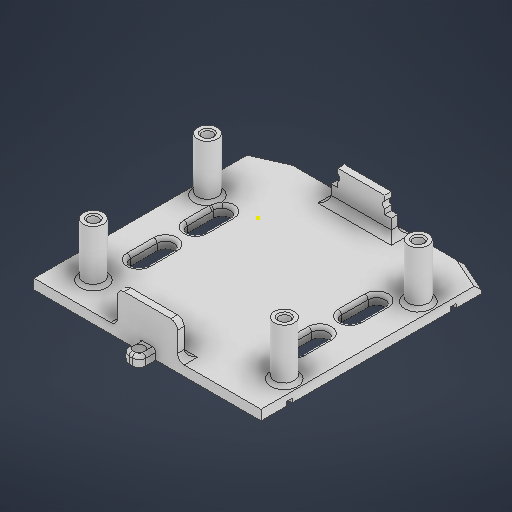
# Autodesk Inventor part: Podstawa2
Saved by Autodesk Inventor 2026 (Build 300175000, 175)
## iProperties
Created: 2025-04-23
Part Number: Podstawa2
Material: Generic
Document SubType Name: Modeling
Designer: isan
Density: 1 g/cm^3
Appearance: Default
Author: isan
Autodesk Inventor part; units mm, degrees
ref_plane "YZ Plane" through (0, 0, 0) normal (1, 0, 0) x (0, 1, 0)
ref_plane "XZ Plane" through (0, 0, 0) normal (0, 1, 0) x (-1, 0, 0)
ref_plane "XY Plane" through (0, 0, 0) normal (0, 0, 1) x (1, 0, 0)
sketch "Sketch2" plane through (0, 0, 0) normal (0, 1, 0) x (-1, 0, 0)
  line L0 (-34, 33) -> (34, 33)
  line L1 (34, 33) -> (34, -33)
  line L2 (34, -33) -> (-34, -33)
  line L3 (-34, -33) -> (-34, 33)
  line L4 (-34, 33) -> (34, -33) construction
  line L5 (34, 33) -> (-34, -33) construction
  point P0 (0, 0)
  dimension "d5" = 66
  dimension "d6" = 68
  constraints: 12 end point, 2 midpoint, 2 parallel, 1 horizontal, 1 perpendicular
  measures "d5" distance of L0.end L1.end
  measures "d6" distance of L1.end L2.end
extrude "Extrusion1" add sketch "Sketch2" along normal blind 3
sketch "Sketch3" plane through (0, 3, 0) normal (0, 1, 0) x (1, 0, 0)
  line L0 (-23.1, 12.5) -> (-23.1, 4.5) construction
  line L1 (-25.6, 12.5) -> (-25.6, 4.5)
  line L2 (-20.6, 4.5) -> (-20.6, 12.5)
  arc A0 (-20.6, 12.5) -> (-25.6, 12.5) centre (-23.1, 12.5) ccw
  arc A1 (-25.6, 4.5) -> (-20.6, 4.5) centre (-23.1, 4.5) ccw
  line L3 (-34, 33) -> (-34, -33) projected
  point P0 (0, 0)
  point P1 (-23.1, 8.5)
  point P2 (-23.1, 15)
  point P3 (-23.1, 2)
  point P4 (-25.6, 8.5)
  dimension "d9" = 13
  dimension "d12" = 2.5
  dimension "d13" = 8.4
  dimension "d14" = 2
  constraints: 8 end point, 6 point on circle, 4 tangent, 2 centre point, 2 midpoint, 1 parallel, 1 vertical
  measures "d9" distance of point (-23.1, 15) point (-23.1, 2)
  measures "d12" radius of A0
  measures "d13" distance from line of L3 point (-25.6, 8.5)
  measures "d14" vertical distance of point (0, 0) point (-23.1, 2)
extrude "Extrusion2" cut sketch "Sketch3" against normal blind 3
mirror "Mirror1" about plane through (0, 0, 0) normal (1, 0, 0) of "Extrusion2"
mirror "Mirror2" about plane through (0, 0, 0) normal (0, 0, 1) of "Extrusion2", "Mirror1"
sketch "Sketch4" plane through (0, 3, 0) normal (0, 1, 0) x (1, 0, 0)
  circle A0 centre (-29.6, 14.557) radius 3
  line L0 (-34, 33) -> (-34, -33) projected
  line L1 (-34, -33) -> (34, -33) projected
  line L2 (34, 33) -> (-34, 33) projected
  circle A1 centre (29.583, -21.6) radius 3
  line L3 (34, -33) -> (34, 33) projected
  circle A2 centre (29.525, 18.595) radius 3
  circle A3 centre (-24.6, -24.6) radius 3
  point P0 (0, 0)
  dimension "d23" = 6
  dimension "d28" = 6
  dimension "d31" = 6
  dimension "d34" = 6
  dimension "d65" = 29.6
  dimension "d66" = 14.557
  dimension "d67" = 29.525
  dimension "d68" = 18.595
  dimension "d69" = 21.6
  dimension "d70" = 29.583
  dimension "d71" = 24.6
  dimension "d72" = 24.6
  constraints: 4 centre point
  measures "d23" diameter of A0
  measures "d28" diameter of A1
  measures "d31" diameter of A2
  measures "d34" diameter of A3
  measures "d65" horizontal distance of point (0, 0) A0.centre
  measures "d66" vertical distance of point (0, 0) A0.centre
  measures "d67" horizontal distance of point (0, 0) A2.centre
  measures "d68" vertical distance of point (0, 0) A2.centre
  measures "d69" vertical distance of point (0, 0) A1.centre
  measures "d70" horizontal distance of point (0, 0) A1.centre
  measures "d71" horizontal distance of A3.centre point (0, 0)
  measures "d72" horizontal distance of point (0, 0) A3.centre
extrude "Extrusion3" add sketch "Sketch4" along normal blind 16 contours A0 | A1 | A2 | A3
sketch "Sketch5" plane through (0, 3, 0) normal (0, 1, 0) x (1, 0, 0)
  line L0 (-9, 33) -> (9, 33)
  line L1 (9, 33) -> (9, 31)
  line L2 (9, 31) -> (-9, 31)
  line L3 (-9, 31) -> (-9, 33)
  line L4 (34, 33) -> (-34, 33) projected
  point P0 (0, 0)
  point P1 (0, 33)
  dimension "d39" = 2
  dimension "d40" = 18
  constraints: 8 end point, 2 midpoint, 2 parallel, 1 collinear, 1 horizontal, 1 perpendicular
  measures "d39" distance of L0.end L1.end
  measures "d40" distance of L0.start L0.end
extrude "Extrusion4" add sketch "Sketch5" along normal blind 10
fillet "Fillet1" radius 2 5 edges at (9, 13, -32) (9, 3, -32) (0, 3, -31) (-9, 13, -32) (-9, 3, -32)
mirror "Mirror3" about plane through (0, 0, 0) normal (0, 0, 1) of "Extrusion4", "Fillet1"
sketch "Sketch6" plane through (-29.6, 19, -14.557) normal (0, 1, 0) x (1, 0, 0)
  point P0 (29.6, -14.557)
sketch "Sketch7" plane through (-29.6, 19, -14.557) normal (0, 1, 0) x (1, 0, 0)
  circle A0 centre (0, 0) radius 1.5
  circle A1 centre (0, 0) radius 3 projected
  point P0 (29.6, -14.557)
  dimension "d44" = 3
  constraints: 1 centre point, 1 coincident
  measures "d44" diameter of A0
extrude "Extrusion5" cut sketch "Sketch7" against normal blind 10 contours A0
sketch "Sketch8" plane through (29.525, 19, -18.595) normal (0, 1, 0) x (1, 0, 0)
  circle A0 centre (0, 0) radius 1.5
  point P0 (-29.525, -18.595)
  dimension "d48" = 3
  constraints: 1 centre point
  measures "d48" diameter of A0
extrude "Extrusion6" cut sketch "Sketch8" against normal blind 10
sketch "Sketch9" plane through (-24.6, 19, 24.6) normal (0, 1, 0) x (1, 0, 0)
  circle A0 centre (0, 0) radius 3 projected
  circle A1 centre (0, 0) radius 1.5
  circle A2 centre (54.183, 3) radius 1.5
  circle A3 centre (54.183, 3) radius 3 projected
  point P0 (24.6, 24.6)
  dimension "d51" = 3
  dimension "d52" = 3
  constraints: 2 centre point, 2 coincident
  measures "d51" diameter of A1
  measures "d52" diameter of A2
extrude "Extrusion7" cut sketch "Sketch9" against normal blind 10 contours A1 | A2
sketch "Sketch11" plane through (0, 0, 0) normal (0, -1, 0) x (1, 0, 0)
  line L0 (-34, 25.4) -> (-13.9, 25.4)
  line L1 (-13.9, 25.4) -> (-13.9, 23.6)
  line L2 (-13.9, 23.6) -> (-34, 23.6)
  line L3 (-34, 23.6) -> (-34, 25.4)
  line L4 (-34, -33) -> (-34, 33) projected
  line L5 (-34, 33) -> (34, 33) projected
  point P0 (0, 0)
  point P1 (-34, 24.5)
  dimension "d60" = 1.8
  dimension "d61" = 20.1
  dimension "d62" = 8.5
  constraints: 8 end point, 2 parallel, 1 collinear, 1 horizontal, 1 midpoint, 1 perpendicular
  measures "d60" distance of L0.end L1.end
  measures "d61" distance of L1.end L2.end
  measures "d62" distance from line of L5 point (-34, 24.5)
extrude "Extrusion9" cut sketch "Sketch11" against normal blind 1.2
mirror "Mirror6" about plane through (0, 0, 0) normal (1, 0, 0) of "Extrusion9"
mirror "Mirror7" about plane through (0, 0, 0) normal (0, 0, 1) of "Extrusion9", "Mirror6"
chamfer "Chamfer3" distance 0.4 angle 45 4 edges at (-31.1, 19, -14.557) (28.025, 19, -18.595) (28.083, 19, 21.6) (-26.1, 19, 24.6)
sketch "Sketch12" plane through (0, 0, 0) normal (0, -1, 0) x (1, 0, 0)
  line L0 (0, -50.2706) -> (0, 0) construction
  line L1 (34, -33) -> (-34, -33) projected
  line L2 (-2.5, 38) -> (2.5, 38)
  line L3 (2.5, 38) -> (2.5, 33)
  line L4 (2.5, 33) -> (-2.5, 33)
  line L5 (-2.5, 33) -> (-2.5, 38)
  line L6 (-2.5, 38) -> (2.5, 33) construction
  line L7 (2.5, 38) -> (-2.5, 33) construction
  circle A0 centre (0, 35.5) radius 1.575
  line L8 (7, 33) -> (-7, 33) projected
  line L9 (0, 41.2812) -> (0, 0) construction
  point P0 (2.5, -33)
  dimension "d82" = 5
  dimension "d83" = 5
  dimension "d84" = 3.15
  constraints: 16 end point, 2 collinear, 2 midpoint, 2 parallel, 1 centre point, 1 coincident, 1 perpendicular, 1 point on line, 1 vertical
  measures "d82" distance of L2.end L3.end
  measures "d83" distance of L2.start L2.end
  measures "d84" diameter of A0
extrude "Extrusion10" add sketch "Sketch12" against normal blind 3
fillet "Fillet2" radius 2 2 edges at (2.5, 1.5, 38) (-2.5, 1.5, 38)
fillet "Fillet3" radius 1 5 edges at (0, 3, 38) (-1.9142, 3, 37.4142) (-2.5, 3, 34.5) (2.5, 3, 34.5) (1.9142, 3, 37.4142)
sketch "Sketch13" plane through (0, 0, 0) normal (0, -1, 0) x (1, 0, 0)
  line L0 (-34, 33) -> (34, 33) projected
  line L1 (25, -37) -> (-25, -37)
  line L2 (-25, -37) -> (-25, -33)
  line L3 (-25, -33) -> (25, -33)
  line L4 (25, -33) -> (25, -37)
  line L5 (25, -37) -> (-25, -33) construction
  line L6 (-25, -37) -> (25, -33) construction
  line L7 (25, -37) -> (34, -33)
  line L8 (-25, -37) -> (-34, -33)
  line L9 (7, -33) -> (-7, -33) projected
  line L10 (0, 0) -> (0, -49.5761) construction
  line L11 (34, -33) -> (-34, -33)
  point P0 (0, -35)
  point P1 (25, -33)
  dimension "d92" = 4
  dimension "d93" = 50
  constraints: 20 end point, 2 coincident, 2 midpoint, 2 parallel, 1 collinear, 1 horizontal, 1 perpendicular, 1 point on line, 1 vertical
  measures "d92" distance of L3.end L1.start
  measures "d93" distance of L1.start L1.end
fillet "Face Fillet5" radius 1 1 edges at (26.583, 3, 21.6)
fillet "Face Fillet6" radius 1 1 edges at (26.525, 3, -18.595)
fillet "Face Fillet7" radius 1 1 edges at (-32.6, 3, -14.557)
fillet "Face Fillet8" radius 1 1 edges at (-27.6, 3, 24.6)
fillet "Fillet4" radius 1 16 edges at (-23.1, 3, -2) (-25.6, 3, -8.5) (-23.1, 3, -15) (-20.6, 3, -8.5) (-23.1, 3, 15) (-25.6, 3, 8.5) (-23.1, 3, 2) (-20.6, 3, 8.5) (23.1, 3, -15) (25.6, 3, -8.5) (23.1, 3, -2) (20.6, 3, -8.5) (23.1, 3, 15) (20.6, 3, 8.5) (23.1, 3, 2) (25.6, 3, 8.5)
extrude "Extrusion14" add sketch "Sketch13" against normal blind 3
chamfer "Chamfer5" distance 2 angle 45 3 edges at (0, 3, -37) (29.5, 3, -35) (-29.5, 3, -35)
fillet "Face Fillet9" radius 2 1 edges at (0, 3, -33)
sketch "Sketch16" plane through (7, 13, -33) normal (0, 0, -1) x (-1, 0, 0)
  line L0 (18, -10) -> (-4, -10) projected
  line L1 (16, -8) -> (16, -2) projected
  line L2 (-2, -10) -> (16, -10)
  line L3 (16, -10) -> (16, -5)
  line L4 (16, -5) -> (-2, -5)
  line L5 (-2, -5) -> (-2, -10)
  line L6 (-2, -8) -> (-2, -2) projected
  line L7 (0, -5) -> (14, -5)
  line L8 (14, -5) -> (14, 0)
  line L9 (14, 0) -> (0, 0)
  line L10 (0, 0) -> (0, -5)
  line L11 (0, 0) -> (14, 0) projected
  line L12 (7, -13) -> (7, 3.9684) construction
  line L13 (0, -5) -> (-8, -5)
  line L14 (-8, -5) -> (-8, 3)
  line L15 (-8, 3) -> (0, 3)
  line L16 (0, 3) -> (0, -5)
  line L17 (14, -5) -> (22, -5)
  line L18 (22, -5) -> (22, 3)
  line L19 (22, 3) -> (14, 3)
  line L20 (14, 3) -> (14, -5)
  arc A0 (0, -3.5) -> (0, -1.5) centre (-0.4583, -2.5) ccw
  arc A1 (14, -1.5) -> (14, -3.5) centre (14.4583, -2.5) ccw
  point P0 (7, 0)
  point P1 (14, -1.5)
  point P2 (14, -3.5)
  point P3 (14, -5)
  point P4 (14, 0)
  point P5 (-2, -5)
  point P6 (0, -3.5)
  point P7 (0, -1.5)
  point P8 (0, 0)
  dimension "d131" = 5
  dimension "d132" = 14
  dimension "d133" = 8
  dimension "d134" = 8
  dimension "d135" = 8
  dimension "d136" = 8
  dimension "d137" = 2
  dimension "d138" = 1.1
  dimension "d140" = 2.5
  dimension "d143" = 1.1
  dimension "d144" = 2
  dimension "d145" = 2.5
  constraints: 34 end point, 8 parallel, 8 point on line, 4 horizontal, 4 perpendicular, 4 point on circle, 2 centre point, 2 collinear, 2 midpoint, 1 vertical
  measures "d131" distance of L4.end L2.start
  measures "d132" distance of L8.end L9.end
  measures "d133" distance of L14.end L15.end
  measures "d134" distance of L13.end L14.end
  measures "d135" distance of L17.end L18.end
  measures "d136" distance of L18.end L19.end
  measures "d137" distance of A0.start A0.end
  measures "d138" radius of A0
  measures "d140" vertical distance of L11.start A0.centre
  measures "d143" radius of A1
  measures "d144" distance of A1.end A1.start
  measures "d145" vertical distance of L11.end A1.centre
extrude "Extrusion15" cut sketch "Sketch16" against normal blind 2 contours L4 L8 L20 L19 L18 L17 | L13 L14 L15 L16 L10 L4 | A1 L8 | L10 A0
body "Solid1"
